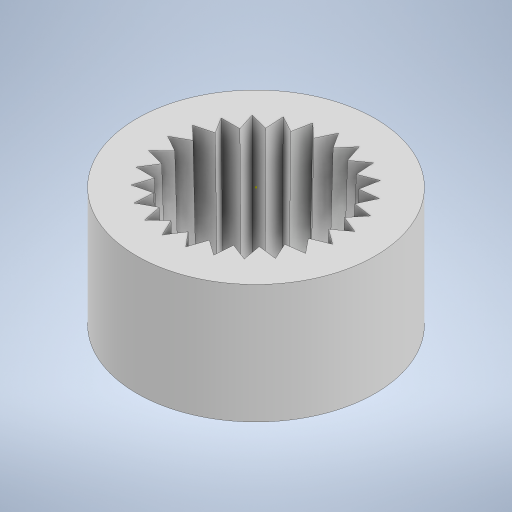
# Autodesk Inventor part: OMG_servo_head(1deg)
Saved by Autodesk Inventor 2023.1 (Build 271208000, 208)
## iProperties
Created: 2026-02-22
Part Number: OMG_servo_head(1deg)
Material: Generic
Document SubType Name: Modeling
Designer: Lars
Density: 1 g/cm^3
Appearance: Default
Author: Lars
Autodesk Inventor part; units mm, degrees
ref_plane "YZ Plane" through (0, 0, 0) normal (1, 0, 0) x (0, 1, 0)
ref_plane "XZ Plane" through (0, 0, 0) normal (0, 1, 0) x (-1, 0, 0)
ref_plane "XY Plane" through (0, 0, 0) normal (0, 0, 1) x (1, 0, 0)
sketch "Sketch1" plane through (0, 0, 0) normal (0, 1, 0) x (-1, 0, 0)
  circle A0 centre (0, 0) radius 2.825 construction
  circle A1 centre (0, 0) radius 2.325 construction
  line L0 (2.825, 0) -> (2.3067, 0.2914)
  line L1 (2.825, 0) -> (2.3067, -0.2914)
  line L2 (2.825, 0) -> (2.325, 0) construction
  line L3 (2.7362, 0.7025) -> (2.1617, 0.8559)
  line L4 (2.7362, 0.7025) -> (2.3067, 0.2914)
  line L5 (2.4756, 1.361) -> (1.881, 1.3666)
  line L6 (2.4756, 1.361) -> (2.1617, 0.8559)
  line L7 (2.0593, 1.9338) -> (1.482, 1.7914)
  line L8 (2.0593, 1.9338) -> (1.881, 1.3666)
  line L9 (1.5137, 2.3852) -> (0.9899, 2.1037)
  line L10 (1.5137, 2.3852) -> (1.482, 1.7914)
  line L11 (0.873, 2.6867) -> (0.4357, 2.2838)
  line L12 (0.873, 2.6867) -> (0.9899, 2.1037)
  line L13 (0.1774, 2.8194) -> (-0.146, 2.3204)
  line L14 (0.1774, 2.8194) -> (0.4357, 2.2838)
  line L15 (-0.5294, 2.775) -> (-0.7185, 2.2112)
  line L16 (-0.5294, 2.775) -> (-0.146, 2.3204)
  line L17 (-1.2028, 2.5561) -> (-1.2458, 1.9631)
  line L18 (-1.2028, 2.5561) -> (-0.7185, 2.2112)
  line L19 (-1.8007, 2.1767) -> (-1.6949, 1.5916)
  line L20 (-1.8007, 2.1767) -> (-1.2458, 1.9631)
  line L21 (-2.2855, 1.6605) -> (-2.0374, 1.1201)
  line L22 (-2.2855, 1.6605) -> (-1.6949, 1.5916)
  line L23 (-2.6266, 1.04) -> (-2.252, 0.5782)
  line L24 (-2.6266, 1.04) -> (-2.0374, 1.1201)
  line L25 (-2.8027, 0.3541) -> (-2.325, 0)
  line L26 (-2.8027, 0.3541) -> (-2.252, 0.5782)
  line L27 (-2.8027, -0.3541) -> (-2.252, -0.5782)
  line L28 (-2.8027, -0.3541) -> (-2.325, 0)
  line L29 (-2.6266, -1.04) -> (-2.0374, -1.1201)
  line L30 (-2.6266, -1.04) -> (-2.252, -0.5782)
  line L31 (-2.2855, -1.6605) -> (-1.6949, -1.5916)
  line L32 (-2.2855, -1.6605) -> (-2.0374, -1.1201)
  line L33 (-1.8007, -2.1767) -> (-1.2458, -1.9631)
  line L34 (-1.8007, -2.1767) -> (-1.6949, -1.5916)
  line L35 (-1.2028, -2.5561) -> (-0.7185, -2.2112)
  line L36 (-1.2028, -2.5561) -> (-1.2458, -1.9631)
  line L37 (-0.5294, -2.775) -> (-0.146, -2.3204)
  line L38 (-0.5294, -2.775) -> (-0.7185, -2.2112)
  line L39 (0.1774, -2.8194) -> (0.4357, -2.2838)
  line L40 (0.1774, -2.8194) -> (-0.146, -2.3204)
  line L41 (0.873, -2.6867) -> (0.9899, -2.1037)
  line L42 (0.873, -2.6867) -> (0.4357, -2.2838)
  line L43 (1.5137, -2.3852) -> (1.482, -1.7914)
  line L44 (1.5137, -2.3852) -> (0.9899, -2.1037)
  line L45 (2.0593, -1.9338) -> (1.881, -1.3666)
  line L46 (2.0593, -1.9338) -> (1.482, -1.7914)
  line L47 (2.4756, -1.361) -> (2.1617, -0.8559)
  line L48 (2.4756, -1.361) -> (1.881, -1.3666)
  line L49 (2.7362, -0.7025) -> (2.3067, -0.2914)
  line L50 (2.7362, -0.7025) -> (2.1617, -0.8559)
  circle A2 centre (0, 0) radius 4
  dimension "d0" = 5.65
  dimension "d1" = 0.5
  dimension "d3" = 0.5
  dimension "d6" = 360
  dimension "d11" = 8
  constraints: 102 end point, 3 coincident, 3 point on circle, 2 centre point, 1 horizontal, 1 horizontal alignment, 129 other
  measures "d3" distance of L0.start L2.end
  measures "d11" diameter of A2
extrude "Extrusion1" add sketch "Sketch1" along normal blind 4 contours L1 L49 L50 L47 L48 L45 L46 L43 L44 L41 L42 L39 L40 L37 L38 L35 L36 L33 L34 L31 L32 L29 L30 L27 L28 L25 L26 L23 L24 L21 L22 L19 L20 L17 L18 L15 L16 L13 L14 L11 L12 L9 L10 L7 L8 L5 L6 L3 L4 L0 | A2
extrude "Extrusion2" cut sketch "Sketch1" along normal blind 4 draft 1 contours L1 L49 L50 L47 L48 L45 L46 L43 L44 L41 L42 L39 L40 L37 L38 L35 L36 L33 L34 L31 L32 L29 L30 L27 L28 L25 L26 L23 L24 L21 L22 L19 L20 L17 L18 L15 L16 L13 L14 L11 L12 L9 L10 L7 L8 L5 L6 L3 L4 L0
sketch "Sketch3" plane through (0, 4, 0) normal (0, 1, 0) x (1, 0, 0)
  point P0 (0, 0)
equation "\"d3\" = d1"
body "Solid1"
